Autodesk Fusion 360 part; units mm, degrees
(part 2 of 25)
sketch "Top SIlkscreen" plane through (0, 0, 0) normal (0, 0, 1) x (1, 0, 0)
  line L0 (55.2958, 9.3303) -> (56.4642, 9.7197)
  arc A0 (55.2878, 9.3544) -> (55.3038, 9.3062) centre (55.2958, 9.3303) ccw
  arc A1 (52.7304, 13.311) -> (52.7812, 13.311) centre (52.7558, 13.311) ccw
  line L1 (56.1721, 9.6224) -> (56.1721, 9.0382)
  arc A2 (56.4722, 9.6956) -> (56.4562, 9.7438) centre (56.4642, 9.7197) ccw
  arc A3 (53.6646, 12.8425) -> (53.6646, 12.7917) centre (53.6646, 12.8171) ccw
  arc A4 (53.9242, 13.2856) -> (53.9242, 13.3364) centre (53.9242, 13.311) ccw
  arc A5 (53.9242, 10.5777) -> (53.9242, 10.6285) centre (53.9242, 10.6031) ccw
  arc A6 (53.6392, 10.1487) -> (53.69, 10.1487) centre (53.6646, 10.1487) ccw
  arc A7 (52.6347, 11.7855) -> (52.6173, 11.7377) centre (52.626, 11.7616) ccw
  arc A8 (53.8988, 12.5575) -> (53.9496, 12.5575) centre (53.9242, 12.5575) ccw
  arc A9 (52.7304, 12.4601) -> (52.7812, 12.4601) centre (52.7558, 12.4601) ccw
  line L2 (53.4049, 10.6031) -> (53.9242, 10.6031)
  arc A10 (53.7619, 12.168) -> (53.9242, 12.5575) centre (53.3757, 12.5575) ccw
  arc A11 (53.8988, 13.6356) -> (53.9496, 13.6356) centre (53.9242, 13.6356) ccw
  arc A12 (52.7638, 14.8408) -> (52.7478, 14.7926) centre (52.7558, 14.8167) ccw
  line L3 (53.9242, 13.6356) -> (53.9242, 13.311)
  arc A13 (52.8532, 12.7522) -> (52.7558, 12.4601) centre (53.2426, 12.4601) ccw
  arc A14 (53.0154, 12.1751) -> (53.0154, 12.2259) centre (53.0154, 12.2005) ccw
  arc A15 (53.6646, 12.8171) -> (53.4374, 12.6873) centre (53.6646, 12.5534) ccw
  line L4 (52.7558, 14.8167) -> (53.9242, 15.2061)
  arc A16 (53.9162, 14.4031) -> (53.9322, 14.4513) centre (53.9242, 14.4272) ccw
  arc A17 (53.69, 10.7978) -> (53.6392, 10.7978) centre (53.6646, 10.7978) ccw
  arc A18 (54.0453, 11.2184) -> (54.0627, 11.2662) centre (54.054, 11.2423) ccw
  arc A19 (53.0804, 13.9347) -> (53.0804, 13.9855) centre (53.0804, 13.9601) ccw
  arc A20 (53.8988, 13.311) -> (53.9496, 13.311) centre (53.9242, 13.311) ccw
  line L5 (56.4642, 8.9408) -> (55.2958, 9.3303)
  arc A21 (52.7812, 13.6356) -> (52.7304, 13.6356) centre (52.7558, 13.6356) ccw
  line L6 (53.9242, 14.4272) -> (52.7558, 14.8167)
  line L7 (53.6321, 15.1088) -> (53.6321, 14.5246)
  arc A22 (52.8735, 12.737) -> (52.8328, 12.7674) centre (52.8531, 12.7522) ccw
  arc A23 (53.0804, 13.9855) -> (53.0804, 13.9347) centre (53.0804, 13.9601) ccw
  arc A24 (55.3038, 9.3544) -> (55.2878, 9.3062) centre (55.2958, 9.3303) ccw
  arc A25 (53.744, 12.186) -> (53.7798, 12.15) centre (53.7619, 12.168) ccw
  arc A26 (53.0154, 12.2005) -> (53.2426, 12.3303) centre (53.0154, 12.4642) ccw
  arc A27 (52.7628, 10.4328) -> (52.7488, 10.3839) centre (52.7558, 10.4084) ccw
  arc A28 (52.7558, 12.4601) -> (53.0154, 12.2005) centre (53.0154, 12.4601) ccw
  line L8 (53.9242, 13.311) -> (52.7558, 13.311)
  arc A29 (53.2203, 12.3424) -> (53.2649, 12.3181) centre (53.2426, 12.3302) ccw
  arc A30 (52.7812, 12.4601) -> (52.7304, 12.4601) centre (52.7558, 12.4601) ccw
  arc A31 (53.4049, 10.6285) -> (53.4049, 10.5777) centre (53.4049, 10.6031) ccw
  arc A32 (53.0154, 12.2259) -> (53.0154, 12.1751) centre (53.0154, 12.2005) ccw
  arc A33 (52.7304, 13.6356) -> (52.7812, 13.6356) centre (52.7558, 13.6356) ccw
  line L9 (53.0804, 13.9601) -> (53.5996, 13.9601)
  arc A34 (53.9496, 12.5575) -> (53.8988, 12.5575) centre (53.9242, 12.5575) ccw
  arc A35 (53.5996, 13.9855) -> (53.5996, 13.9347) centre (53.5996, 13.9601) ccw
  arc A36 (53.5996, 13.9347) -> (53.5996, 13.9855) centre (53.5996, 13.9601) ccw
  line L10 (53.4374, 12.6873) -> (53.2426, 12.3303)
  arc A37 (53.0804, 13.9601) -> (52.7558, 13.6356) centre (53.0804, 13.6355) ccw
  arc A38 (53.9242, 13.6356) -> (53.5996, 13.9601) centre (53.5996, 13.6355) ccw
  arc A39 (53.9242, 12.5575) -> (53.6646, 12.8171) centre (53.6646, 12.5575) ccw
  arc A40 (53.2645, 12.3174) -> (53.2208, 12.3432) centre (53.2427, 12.3303) ccw
  arc A41 (53.4155, 12.7002) -> (53.4593, 12.6744) centre (53.4374, 12.6873) ccw
  arc A42 (53.4597, 12.6751) -> (53.4151, 12.6995) centre (53.4374, 12.6873) ccw
  arc A43 (53.9322, 15.182) -> (53.9162, 15.2302) centre (53.9242, 15.2061) ccw
  arc A44 (56.4562, 8.9167) -> (56.4722, 8.9649) centre (56.4642, 8.9408) ccw
  arc A45 (53.6646, 12.7917) -> (53.6646, 12.8425) centre (53.6646, 12.8171) ccw
  arc A46 (52.7478, 14.8408) -> (52.7638, 14.7926) centre (52.7558, 14.8167) ccw
  line L11 (54.054, 11.2423) -> (52.626, 11.7616)
  arc A47 (53.6575, 15.1088) -> (53.6067, 15.1088) centre (53.6321, 15.1088) ccw
  line L12 (52.7558, 13.311) -> (52.7558, 13.6356)
  arc A48 (52.7558, 13.3364) -> (52.7558, 13.2856) centre (52.7558, 13.311) ccw
  arc A49 (53.6067, 14.5246) -> (53.6575, 14.5246) centre (53.6321, 14.5246) ccw
  arc A50 (53.9496, 13.6356) -> (53.8988, 13.6356) centre (53.9242, 13.6356) ccw
  arc A51 (55.3212, 12.4601) -> (55.2704, 12.4601) centre (55.2958, 12.4601) ccw
  arc A52 (56.4642, 10.5382) -> (56.2046, 10.7978) centre (56.2046, 10.5382) ccw
  arc A53 (56.2046, 10.7724) -> (56.2046, 10.8232) centre (56.2046, 10.7978) ccw
  arc A54 (41.0619, 54.9233) -> (41.2242, 55.1504) centre (40.9841, 55.1504) ccw
  arc A55 (56.2046, 12.8425) -> (56.2046, 12.7917) centre (56.2046, 12.8171) ccw
  arc A56 (41.0537, 54.9473) -> (41.0702, 54.8992) centre (41.062, 54.9233) ccw
  line L13 (56.4642, 10.1487) -> (56.4642, 10.5382)
  arc A57 (56.4388, 12.5575) -> (56.4896, 12.5575) centre (56.4642, 12.5575) ccw
  arc A58 (41.1988, 55.1504) -> (41.2496, 55.1504) centre (41.2242, 55.1504) ccw
  arc A59 (55.2958, 10.1741) -> (55.2958, 10.1233) centre (55.2958, 10.1487) ccw
  arc A60 (40.64, 54.8513) -> (40.64, 54.8005) centre (40.64, 54.8259) ccw
  arc A61 (56.0747, 10.7724) -> (56.0747, 10.8232) centre (56.0747, 10.7978) ccw
  arc A62 (41.2242, 55.1504) -> (41.0619, 55.3776) centre (40.984, 55.1504) ccw
  arc A63 (41.0508, 55.3548) -> (41.0731, 55.4005) centre (41.0619, 55.3777) ccw
  arc A64 (55.7897, 10.1487) -> (55.8405, 10.1487) centre (55.8151, 10.1487) ccw
  arc A65 (55.3212, 10.7978) -> (55.2704, 10.7978) centre (55.2958, 10.7978) ccw
  arc A66 (56.4388, 10.1487) -> (56.4896, 10.1487) centre (56.4642, 10.1487) ccw
  line L14 (55.2958, 10.1487) -> (55.2958, 10.7978)
  arc A67 (56.4642, 12.5575) -> (56.2046, 12.8171) centre (56.2046, 12.5575) ccw
  arc A68 (34.8822, 28.7456) -> (34.8662, 28.7938) centre (34.8742, 28.7697) ccw
  arc A69 (40.64, 55.5004) -> (40.64, 55.4496) centre (40.64, 55.475) ccw
  arc A70 (56.4896, 10.5382) -> (56.4388, 10.5382) centre (56.4642, 10.5382) ccw
  arc A71 (56.3019, 12.168) -> (56.4642, 12.5575) centre (55.9157, 12.5575) ccw
  arc A72 (55.1747, 11.7855) -> (55.1573, 11.7377) centre (55.166, 11.7616) ccw
  arc A73 (55.5554, 12.1751) -> (55.5554, 12.2259) centre (55.5554, 12.2005) ccw
  arc A74 (56.2046, 10.8232) -> (56.2046, 10.7724) centre (56.2046, 10.7978) ccw
  arc A75 (55.8405, 10.5382) -> (55.7897, 10.5382) centre (55.8151, 10.5382) ccw
  arc A76 (41.0702, 55.4017) -> (41.0537, 55.3536) centre (41.0619, 55.3777) ccw
  arc A77 (55.8151, 10.1233) -> (55.8151, 10.1741) centre (55.8151, 10.1487) ccw
  line L15 (56.594, 11.2423) -> (55.166, 11.7616)
  line L16 (55.8151, 10.5382) -> (55.8151, 10.1487)
  arc A78 (40.9487, 54.871) -> (40.9804, 54.9106) centre (40.9646, 54.8908) ccw
  line L17 (40.9646, 54.8908) -> (40.3154, 55.4101)
  arc A79 (41.0619, 55.3776) -> (40.64, 55.475) centre (40.6399, 54.5123) ccw
  arc A80 (40.3313, 55.4299) -> (40.2996, 55.3903) centre (40.3154, 55.4101) ccw
  line L18 (43.7642, 52.5018) -> (42.5958, 52.5018)
  line L19 (42.5958, 52.5018) -> (42.5958, 52.8264)
  arc A81 (56.0747, 10.8232) -> (56.0747, 10.7724) centre (56.0747, 10.7978) ccw
  arc A82 (55.2704, 10.1487) -> (55.3212, 10.1487) centre (55.2958, 10.1487) ccw
  line L20 (56.2046, 10.7978) -> (56.0747, 10.7978)
  arc A83 (56.1975, 9.6224) -> (56.1467, 9.6224) centre (56.1721, 9.6224) ccw
  arc A84 (56.0747, 10.7978) -> (55.8151, 10.5382) centre (56.0747, 10.5382) ccw
  line L21 (55.8151, 10.1487) -> (55.2958, 10.1487)
  arc A85 (55.2958, 12.4601) -> (55.5554, 12.2005) centre (55.5554, 12.4601) ccw
  arc A86 (55.3932, 12.7522) -> (55.2958, 12.4601) centre (55.7826, 12.4601) ccw
  arc A87 (56.284, 12.186) -> (56.3198, 12.15) centre (56.3019, 12.168) ccw
  line L22 (26.6051, 29.6644) -> (26.6051, 29.2749)
  arc A88 (56.4896, 12.5575) -> (56.4388, 12.5575) centre (56.4642, 12.5575) ccw
  arc A89 (40.64, 55.4496) -> (40.64, 55.5004) centre (40.64, 55.475) ccw
  arc A90 (40.2069, 55.4005) -> (40.2292, 55.3548) centre (40.218, 55.3777) ccw
  arc A91 (41.0731, 54.9004) -> (41.0508, 54.9461) centre (41.062, 54.9233) ccw
  arc A92 (56.4388, 10.5382) -> (56.4896, 10.5382) centre (56.4642, 10.5382) ccw
  line L23 (43.9972, 30.4165) -> (44.6322, 30.4165)
  arc A93 (40.0304, 55.1504) -> (40.0812, 55.1504) centre (40.0558, 55.1504) ccw
  arc A94 (41.2496, 55.1504) -> (41.1988, 55.1504) centre (41.2242, 55.1504) ccw
  line L24 (29.1451, 28.4452) -> (29.1451, 28.6399)
  arc A95 (56.5853, 11.2184) -> (56.6027, 11.2662) centre (56.594, 11.2423) ccw
  arc A96 (47.9679, 10.7724) -> (47.9679, 10.8232) centre (47.9679, 10.7978) ccw
  line L25 (26.6051, 29.2749) -> (26.0858, 29.2749)
  arc A97 (40.64, 55.475) -> (40.2181, 55.3776) centre (40.6401, 54.5123) ccw
  arc A98 (56.1467, 9.0382) -> (56.1975, 9.0382) centre (56.1721, 9.0382) ccw
  arc A99 (40.64, 54.8259) -> (41.0619, 54.9233) centre (40.6399, 55.7886) ccw
  arc A100 (55.7897, 10.5382) -> (55.8405, 10.5382) centre (55.8151, 10.5382) ccw
  arc A101 (45.8526, 54.3066) -> (45.8526, 54.3574) centre (45.8526, 54.332) ccw
  arc A102 (42.9204, 53.1509) -> (42.5958, 52.8264) centre (42.9204, 52.8263) ccw
  line L26 (43.7642, 52.8264) -> (43.7642, 52.5018)
  arc A103 (45.8526, 53.7083) -> (45.8526, 53.6575) centre (45.8526, 53.6829) ccw
  arc A104 (45.8526, 53.1763) -> (45.8526, 53.1255) centre (45.8526, 53.1509) ccw
  arc A105 (45.8526, 54.3574) -> (45.8526, 54.3066) centre (45.8526, 54.332) ccw
  arc A106 (45.2684, 53.7478) -> (45.2684, 54.2671) centre (45.2684, 54.0075) ccw
  arc A107 (43.7388, 52.8264) -> (43.7896, 52.8264) centre (43.7642, 52.8264) ccw
  arc A108 (45.3334, 53.1255) -> (45.3334, 53.1763) centre (45.3334, 53.1509) ccw
  arc A109 (44.9834, 52.5018) -> (45.0342, 52.5018) centre (45.0088, 52.5018) ccw
  arc A110 (45.2684, 54.2925) -> (45.2684, 54.2417) centre (45.2684, 54.2671) ccw
  arc A111 (45.2684, 53.7732) -> (45.2684, 53.7224) centre (45.2684, 53.7478) ccw
  arc A112 (42.9853, 53.6829) -> (43.2449, 53.9425) centre (42.9853, 53.9425) ccw
  arc A113 (42.9204, 53.6575) -> (42.9204, 53.7083) centre (42.9204, 53.6829) ccw
  arc A114 (42.9204, 54.3066) -> (42.9204, 54.3574) centre (42.9204, 54.332) ccw
  arc A115 (43.2449, 54.3066) -> (43.2449, 54.3574) centre (43.2449, 54.332) ccw
  arc A116 (43.2449, 54.3574) -> (43.2449, 54.3066) centre (43.2449, 54.332) ccw
  arc A117 (42.9204, 53.7083) -> (42.9204, 53.6575) centre (42.9204, 53.6829) ccw
  arc A118 (42.9853, 53.6575) -> (42.9853, 53.7083) centre (42.9853, 53.6829) ccw
  arc A119 (42.9204, 53.1763) -> (42.9204, 53.1255) centre (42.9204, 53.1509) ccw
  arc A120 (43.2703, 53.9425) -> (43.2195, 53.9425) centre (43.2449, 53.9425) ccw
  arc A121 (42.5704, 52.8264) -> (42.6212, 52.8264) centre (42.5958, 52.8264) ccw
  arc A122 (43.2703, 54.332) -> (43.2195, 54.332) centre (43.2449, 54.332) ccw
  line L27 (42.9853, 53.6829) -> (42.9204, 53.6829)
  line L28 (42.9204, 54.332) -> (43.2449, 54.332)
  arc A123 (43.7642, 53.8127) -> (43.2449, 54.332) centre (43.2449, 53.8127) ccw
  arc A124 (46.1772, 52.4764) -> (46.1772, 52.5272) centre (46.1772, 52.5018) ccw
  arc A125 (45.0342, 52.8264) -> (44.9834, 52.8264) centre (45.0088, 52.8264) ccw
  line L29 (42.9204, 53.1509) -> (43.4396, 53.1509)
  arc A126 (45.0088, 52.5272) -> (45.0088, 52.4764) centre (45.0088, 52.5018) ccw
  line L30 (45.0088, 52.5018) -> (45.0088, 52.8264)
  line L31 (45.3334, 53.1509) -> (45.8526, 53.1509)
  arc A127 (42.9204, 54.332) -> (42.9204, 53.6829) centre (42.9204, 54.0074) ccw
  arc A128 (43.7388, 52.5018) -> (43.7896, 52.5018) centre (43.7642, 52.5018) ccw
  arc A129 (45.3334, 53.1763) -> (45.3334, 53.1255) centre (45.3334, 53.1509) ccw
  arc A130 (46.1518, 52.8264) -> (46.2026, 52.8264) centre (46.1772, 52.8264) ccw
  arc A131 (43.7642, 52.8264) -> (43.4396, 53.1509) centre (43.4396, 52.8263) ccw
  line L32 (46.1772, 52.8264) -> (46.1772, 52.5018)
  arc A132 (45.3334, 53.1509) -> (45.0088, 52.8264) centre (45.3334, 52.8263) ccw
  arc A133 (45.8526, 53.6575) -> (45.8526, 53.7083) centre (45.8526, 53.6829) ccw
  arc A134 (43.7896, 52.8264) -> (43.7388, 52.8264) centre (43.7642, 52.8264) ccw
  arc A135 (46.1772, 52.8264) -> (45.8526, 53.1509) centre (45.8526, 52.8263) ccw
  arc A136 (42.9853, 53.7083) -> (42.9853, 53.6575) centre (42.9853, 53.6829) ccw
  arc A137 (45.2684, 54.2417) -> (45.2684, 54.2925) centre (45.2684, 54.2671) ccw
  arc A138 (45.2684, 53.7224) -> (45.2684, 53.7732) centre (45.2684, 53.7478) ccw
  arc A139 (42.5704, 52.5018) -> (42.6212, 52.5018) centre (42.5958, 52.5018) ccw
  arc A140 (43.4396, 53.1255) -> (43.4396, 53.1763) centre (43.4396, 53.1509) ccw
  arc A141 (43.2195, 53.9425) -> (43.2703, 53.9425) centre (43.2449, 53.9425) ccw
  line L33 (46.1772, 52.5018) -> (45.0088, 52.5018)
  arc A142 (45.8526, 53.1255) -> (45.8526, 53.1763) centre (45.8526, 53.1509) ccw
  arc A143 (42.5958, 52.5272) -> (42.5958, 52.4764) centre (42.5958, 52.5018) ccw
  arc A144 (42.9204, 53.1255) -> (42.9204, 53.1763) centre (42.9204, 53.1509) ccw
  arc A145 (42.9204, 54.3574) -> (42.9204, 54.3066) centre (42.9204, 54.332) ccw
  arc A146 (46.1518, 52.5018) -> (46.2026, 52.5018) centre (46.1772, 52.5018) ccw
  arc A147 (42.6212, 52.8264) -> (42.5704, 52.8264) centre (42.5958, 52.8264) ccw
  arc A148 (43.7388, 53.8127) -> (43.7896, 53.8127) centre (43.7642, 53.8127) ccw
  arc A149 (43.4396, 53.1763) -> (43.4396, 53.1255) centre (43.4396, 53.1509) ccw
  line L34 (43.2449, 54.332) -> (43.2449, 53.9425)
  arc A150 (44.9834, 52.8264) -> (45.0342, 52.8264) centre (45.0088, 52.8264) ccw
  arc A151 (43.7642, 52.4764) -> (43.7642, 52.5272) centre (43.7642, 52.5018) ccw
  arc A152 (45.8526, 53.6829) -> (45.8526, 54.332) centre (45.8526, 54.0074) ccw
  arc A153 (46.2026, 52.8264) -> (46.1518, 52.8264) centre (46.1772, 52.8264) ccw
  arc A154 (45.8526, 54.332) -> (45.8526, 53.6829) centre (45.8526, 54.0074) ccw
  arc A155 (45.2684, 54.2671) -> (45.2684, 53.7478) centre (45.2684, 54.0075) ccw
  arc A156 (51.0596, 54.3066) -> (51.0596, 54.3574) centre (51.0596, 54.332) ccw
  arc A157 (48.0004, 53.189) -> (48.0004, 53.2398) centre (48.0004, 53.2144) ccw
  line L35 (47.6758, 53.7464) -> (47.6758, 54.3955)
  arc A158 (50.5404, 53.1509) -> (50.2158, 52.8264) centre (50.5404, 52.8263) ccw
  arc A159 (47.6758, 52.5907) -> (47.6758, 52.5399) centre (47.6758, 52.5653) ccw
  arc A160 (50.2412, 54.2022) -> (50.1904, 54.2022) centre (50.2158, 54.2022) ccw
  arc A161 (51.0596, 53.6575) -> (51.0596, 53.7083) centre (51.0596, 53.6829) ccw
  arc A162 (47.6504, 53.7464) -> (47.7012, 53.7464) centre (47.6758, 53.7464) ccw
  line L36 (53.9242, 52.5018) -> (52.7558, 52.5018)
  arc A163 (47.7012, 52.8899) -> (47.6504, 52.8899) centre (47.6758, 52.8899) ccw
  arc A164 (47.6504, 52.5653) -> (47.7012, 52.5653) centre (47.6758, 52.5653) ccw
  arc A165 (48.5196, 53.189) -> (48.5196, 53.2398) centre (48.5196, 53.2144) ccw
  arc A166 (48.8188, 52.8899) -> (48.8696, 52.8899) centre (48.8442, 52.8899) ccw
  arc A167 (50.5404, 53.1763) -> (50.5404, 53.1255) centre (50.5404, 53.1509) ccw
  arc A168 (48.0004, 53.2144) -> (47.6758, 52.8899) centre (48.0004, 52.8898) ccw
  line L37 (51.3842, 52.8264) -> (51.3842, 52.5018)
  arc A169 (51.0596, 53.1763) -> (51.0596, 53.1255) centre (51.0596, 53.1509) ccw
  arc A170 (51.3588, 52.5018) -> (51.4096, 52.5018) centre (51.3842, 52.5018) ccw
  arc A171 (51.3842, 52.8264) -> (51.0596, 53.1509) centre (51.0596, 52.8263) ccw
  arc A172 (47.6826, 54.42) -> (47.669, 54.371) centre (47.6758, 54.3955) ccw
  arc A173 (50.1904, 52.8264) -> (50.2412, 52.8264) centre (50.2158, 52.8264) ccw
  line L38 (47.6758, 54.3955) -> (48.8442, 54.071)
  line L39 (50.5404, 53.1509) -> (51.0596, 53.1509)
  arc A174 (51.0596, 53.1255) -> (51.0596, 53.1763) centre (51.0596, 53.1509) ccw
  arc A175 (51.4096, 52.8264) -> (51.3588, 52.8264) centre (51.3842, 52.8264) ccw
  line L40 (48.8442, 52.8899) -> (48.8442, 52.5653)
  arc A176 (50.9947, 54.332) -> (50.7351, 54.0724) centre (50.9947, 54.0724) ccw
  arc A177 (50.7605, 54.0724) -> (50.7097, 54.0724) centre (50.7351, 54.0724) ccw
  arc A178 (47.7012, 54.3955) -> (47.6504, 54.3955) centre (47.6758, 54.3955) ccw
  arc A179 (50.9947, 54.3066) -> (50.9947, 54.3574) centre (50.9947, 54.332) ccw
  line L41 (50.9947, 54.332) -> (51.0596, 54.332)
  arc A180 (51.0596, 53.6829) -> (51.0596, 54.332) centre (51.0596, 54.0074) ccw
  arc A181 (47.6504, 52.8899) -> (47.7012, 52.8899) centre (47.6758, 52.8899) ccw
  line L42 (48.0004, 53.2144) -> (48.5196, 53.2144)
  arc A182 (48.5196, 53.2398) -> (48.5196, 53.189) centre (48.5196, 53.2144) ccw
  arc A183 (51.3842, 52.4764) -> (51.3842, 52.5272) centre (51.3842, 52.5018) ccw
  arc A184 (48.8374, 54.0465) -> (48.851, 54.0954) centre (48.8442, 54.0709) ccw
  arc A185 (51.3588, 52.8264) -> (51.4096, 52.8264) centre (51.3842, 52.8264) ccw
  arc A186 (48.8442, 52.8899) -> (48.5196, 53.2144) centre (48.5196, 52.8898) ccw
  arc A187 (51.0596, 54.3574) -> (51.0596, 54.3066) centre (51.0596, 54.332) ccw
  line L43 (50.2158, 52.5018) -> (50.2158, 52.8264)
  arc A188 (50.7351, 53.7083) -> (50.7351, 53.6575) centre (50.7351, 53.6829) ccw
  arc A189 (50.5404, 53.1255) -> (50.5404, 53.1763) centre (50.5404, 53.1509) ccw
  arc A190 (50.7351, 53.6575) -> (50.7351, 53.7083) centre (50.7351, 53.6829) ccw
  arc A191 (50.2158, 54.2022) -> (50.7351, 53.6829) centre (50.7351, 54.2022) ccw
  arc A192 (47.6758, 53.7718) -> (47.6758, 53.721) centre (47.6758, 53.7464) ccw
  arc A193 (50.2158, 52.5272) -> (50.2158, 52.4764) centre (50.2158, 52.5018) ccw
  arc A194 (50.1904, 52.5018) -> (50.2412, 52.5018) centre (50.2158, 52.5018) ccw
  arc A195 (50.7097, 54.0724) -> (50.7605, 54.0724) centre (50.7351, 54.0724) ccw
  arc A196 (50.9947, 54.3574) -> (50.9947, 54.3066) centre (50.9947, 54.332) ccw
  line L44 (47.6758, 52.5653) -> (47.6758, 52.8899)
  arc A197 (48.8696, 52.8899) -> (48.8188, 52.8899) centre (48.8442, 52.8899) ccw
  arc A198 (48.8442, 52.5399) -> (48.8442, 52.5907) centre (48.8442, 52.5653) ccw
  arc A199 (47.8056, 53.721) -> (47.8056, 53.7718) centre (47.8056, 53.7464) ccw
  line L45 (47.8056, 53.7464) -> (47.6758, 53.7464)
  arc A200 (48.0004, 53.2398) -> (48.0004, 53.189) centre (48.0004, 53.2144) ccw
  line L46 (51.3842, 52.5018) -> (50.2158, 52.5018)
  line L47 (48.8442, 52.5653) -> (47.6758, 52.5653)
  arc A201 (50.2412, 52.8264) -> (50.1904, 52.8264) centre (50.2158, 52.8264) ccw
  arc A202 (48.8188, 52.5653) -> (48.8696, 52.5653) centre (48.8442, 52.5653) ccw
  arc A203 (50.7097, 53.6829) -> (50.7605, 53.6829) centre (50.7351, 53.6829) ccw
  line L48 (50.7351, 53.6829) -> (50.7351, 54.0724)
  arc A204 (51.0596, 53.7083) -> (51.0596, 53.6575) centre (51.0596, 53.6829) ccw
  line L49 (51.0596, 53.6829) -> (50.7351, 53.6829)
  line L50 (56.4642, 52.5018) -> (55.2958, 52.5018)
  arc A205 (40.2263, 55.3536) -> (40.2098, 55.4017) centre (40.2181, 55.3776) ccw
  arc A206 (53.5996, 53.1255) -> (53.5996, 53.1763) centre (53.5996, 53.1509) ccw
  arc A207 (53.9496, 52.8264) -> (53.8988, 52.8264) centre (53.9242, 52.8264) ccw
  arc A208 (54.6885, 2.4638) -> (54.6885, 2.5146) centre (54.6885, 2.4892) ccw
  arc A209 (55.2704, 52.5018) -> (55.3212, 52.5018) centre (55.2958, 52.5018) ccw
  arc A210 (55.6204, 53.1255) -> (55.6204, 53.1763) centre (55.6204, 53.1509) ccw
  arc A211 (53.0804, 53.1509) -> (52.7558, 52.8264) centre (53.0804, 52.8263) ccw
  arc A212 (56.4388, 52.8264) -> (56.4896, 52.8264) centre (56.4642, 52.8264) ccw
  line L51 (52.7558, 52.5018) -> (52.7558, 52.8264)
  arc A213 (53.9242, 52.4764) -> (53.9242, 52.5272) centre (53.9242, 52.5018) ccw
  line L52 (26.0858, 30.353) -> (27.2542, 30.7425)
  arc A214 (54.4542, 1.5804) -> (54.4034, 1.5804) centre (54.4288, 1.5804) ccw
  line L53 (53.6646, 54.332) -> (53.5347, 54.332)
  arc A215 (26.8647, 29.8986) -> (26.8647, 29.9494) centre (26.8647, 29.924) ccw
  arc A216 (53.6646, 54.3066) -> (53.6646, 54.3574) centre (53.6646, 54.332) ccw
  arc A217 (53.5347, 54.3574) -> (53.5347, 54.3066) centre (53.5347, 54.332) ccw
  arc A218 (53.5347, 54.332) -> (53.2751, 54.0724) centre (53.5347, 54.0724) ccw
  arc A219 (53.5347, 54.3066) -> (53.5347, 54.3574) centre (53.5347, 54.332) ccw
  arc A220 (53.5996, 53.1763) -> (53.5996, 53.1255) centre (53.5996, 53.1509) ccw
  arc A221 (53.8988, 54.0724) -> (53.9496, 54.0724) centre (53.9242, 54.0724) ccw
  arc A222 (52.7304, 52.8264) -> (52.7812, 52.8264) centre (52.7558, 52.8264) ccw
  arc A223 (53.9242, 54.0724) -> (53.6646, 54.332) centre (53.6646, 54.0724) ccw
  arc A224 (53.8988, 53.6829) -> (53.9496, 53.6829) centre (53.9242, 53.6829) ccw
  arc A225 (52.7558, 53.7083) -> (52.7558, 53.6575) centre (52.7558, 53.6829) ccw
  arc A226 (34.8662, 27.9667) -> (34.8822, 28.0149) centre (34.8742, 27.9908) ccw
  arc A227 (53.2497, 53.6829) -> (53.3005, 53.6829) centre (53.2751, 53.6829) ccw
  arc A228 (53.3005, 54.0724) -> (53.2497, 54.0724) centre (53.2751, 54.0724) ccw
  arc A229 (53.0804, 53.1255) -> (53.0804, 53.1763) centre (53.0804, 53.1509) ccw
  arc A230 (53.2751, 53.6575) -> (53.2751, 53.7083) centre (53.2751, 53.6829) ccw
  arc A231 (52.7812, 54.332) -> (52.7304, 54.332) centre (52.7558, 54.332) ccw
  arc A232 (56.4642, 52.4764) -> (56.4642, 52.5272) centre (56.4642, 52.5018) ccw
  arc A233 (51.1246, 29.8986) -> (51.1246, 29.9494) centre (51.1246, 29.924) ccw
  line L54 (29.7942, 28.6399) -> (29.7942, 28.2504)
  arc A234 (52.7812, 52.8264) -> (52.7304, 52.8264) centre (52.7558, 52.8264) ccw
  arc A235 (53.8988, 52.5018) -> (53.9496, 52.5018) centre (53.9242, 52.5018) ccw
  line L55 (53.9242, 52.8264) -> (53.9242, 52.5018)
  arc A236 (53.2497, 54.0724) -> (53.3005, 54.0724) centre (53.2751, 54.0724) ccw
  arc A237 (54.9481, 2.4638) -> (54.9481, 2.5146) centre (54.9481, 2.4892) ccw
  arc A238 (55.3212, 52.8264) -> (55.2704, 52.8264) centre (55.2958, 52.8264) ccw
  arc A239 (53.0804, 53.1763) -> (53.0804, 53.1255) centre (53.0804, 53.1509) ccw
  arc A240 (55.2958, 52.5272) -> (55.2958, 52.4764) centre (55.2958, 52.5018) ccw
  arc A241 (53.6646, 54.3574) -> (53.6646, 54.3066) centre (53.6646, 54.332) ccw
  arc A242 (55.6204, 53.1509) -> (55.2958, 52.8264) centre (55.6204, 52.8263) ccw
  arc A243 (55.2704, 52.8264) -> (55.3212, 52.8264) centre (55.2958, 52.8264) ccw
  arc A244 (52.7304, 52.5018) -> (52.7812, 52.5018) centre (52.7558, 52.5018) ccw
  arc A245 (53.8988, 52.8264) -> (53.9496, 52.8264) centre (53.9242, 52.8264) ccw
  arc A246 (53.9496, 54.0724) -> (53.8988, 54.0724) centre (53.9242, 54.0724) ccw
  line L56 (52.7558, 53.6829) -> (52.7558, 54.332)
  arc A247 (52.7304, 53.6829) -> (52.7812, 53.6829) centre (52.7558, 53.6829) ccw
  arc A248 (52.7558, 52.5272) -> (52.7558, 52.4764) centre (52.7558, 52.5018) ccw
  arc A249 (28.8854, 28.0162) -> (28.8854, 27.9654) centre (28.8854, 27.9908) ccw
  arc A250 (26.0778, 30.3771) -> (26.0938, 30.3289) centre (26.0858, 30.353) ccw
  line L57 (53.0804, 53.1509) -> (53.5996, 53.1509)
  arc A251 (26.0604, 29.2749) -> (26.1112, 29.2749) centre (26.0858, 29.2749) ccw
  arc A252 (33.7138, 28.4044) -> (33.6978, 28.3562) centre (33.7058, 28.3803) ccw
  arc A253 (53.9242, 52.8264) -> (53.5996, 53.1509) centre (53.5996, 52.8263) ccw
  line L58 (53.9242, 53.6829) -> (53.9242, 54.0724)
  line L59 (53.2751, 54.0724) -> (53.2751, 53.6829)
  arc A254 (29.8196, 28.6399) -> (29.7688, 28.6399) centre (29.7942, 28.6399) ccw
  line L60 (53.2751, 53.6829) -> (52.7558, 53.6829)
  line L61 (55.6204, 53.1509) -> (56.1396, 53.1509)
  line L62 (55.2958, 52.5018) -> (55.2958, 52.8264)
  arc A255 (56.1396, 53.1255) -> (56.1396, 53.1763) centre (56.1396, 53.1509) ccw
  arc A256 (61.5442, 52.8264) -> (61.2196, 53.1509) centre (61.2196, 52.8263) ccw
  arc A257 (56.23, 54.332) -> (56.1792, 54.332) centre (56.2046, 54.332) ccw
  arc A258 (58.1604, 53.1763) -> (58.1604, 53.1255) centre (58.1604, 53.1509) ccw
  line L63 (59.0042, 53.6829) -> (59.0042, 54.0075)
  arc A259 (59.0042, 54.0075) -> (58.3551, 54.0075) centre (58.6797, 54.0075) ccw
  arc A260 (55.3028, 53.967) -> (55.2888, 53.9181) centre (55.2958, 53.9426) ccw
  arc A261 (58.1604, 53.1509) -> (57.8358, 52.8264) centre (58.1604, 52.8263) ccw
  line L64 (56.2046, 53.6829) -> (56.2046, 54.332)
  arc A262 (58.3297, 54.0075) -> (58.3805, 54.0075) centre (58.3551, 54.0075) ccw
  arc A263 (57.8612, 52.8264) -> (57.8104, 52.8264) centre (57.8358, 52.8264) ccw
  arc A264 (57.8104, 53.6829) -> (57.8612, 53.6829) centre (57.8358, 53.6829) ccw
  arc A265 (56.1792, 53.6829) -> (56.23, 53.6829) centre (56.2046, 53.6829) ccw
  arc A266 (58.1604, 53.1255) -> (58.1604, 53.1763) centre (58.1604, 53.1509) ccw
  arc A267 (58.3551, 54.0724) -> (57.8358, 54.0724) centre (58.0954, 54.0724) ccw
  arc A268 (56.4896, 52.8264) -> (56.4388, 52.8264) centre (56.4642, 52.8264) ccw
  arc A269 (58.3297, 54.0724) -> (58.3805, 54.0724) centre (58.3551, 54.0724) ccw
  arc A270 (59.0296, 52.8264) -> (58.9788, 52.8264) centre (59.0042, 52.8264) ccw
  arc A271 (60.3758, 52.5272) -> (60.3758, 52.4764) centre (60.3758, 52.5018) ccw
  arc A272 (61.5442, 52.4764) -> (61.5442, 52.5272) centre (61.5442, 52.5018) ccw
  line L65 (61.5442, 52.5018) -> (60.3758, 52.5018)
  arc A273 (58.3297, 53.8127) -> (58.3805, 53.8127) centre (58.3551, 53.8127) ccw
  arc A274 (60.4012, 52.8264) -> (60.3504, 52.8264) centre (60.3758, 52.8264) ccw
  line L66 (59.0042, 52.5018) -> (57.8358, 52.5018)
  line L67 (55.9449, 54.1373) -> (56.4642, 54.1373)
  line L68 (59.0042, 52.8264) -> (59.0042, 52.5018)
  arc A275 (58.9788, 53.6829) -> (59.0296, 53.6829) centre (59.0042, 53.6829) ccw
  arc A276 (60.7004, 53.1509) -> (60.3758, 52.8264) centre (60.7004, 52.8263) ccw
  arc A277 (57.8104, 52.5018) -> (57.8612, 52.5018) centre (57.8358, 52.5018) ccw
  line L69 (60.7004, 53.1509) -> (61.2196, 53.1509)
  arc A278 (59.0042, 52.8264) -> (58.6796, 53.1509) centre (58.6796, 52.8263) ccw
  arc A279 (58.9788, 52.8264) -> (59.0296, 52.8264) centre (59.0042, 52.8264) ccw
  arc A280 (60.3504, 52.8264) -> (60.4012, 52.8264) centre (60.3758, 52.8264) ccw
  arc A281 (57.8612, 54.0724) -> (57.8104, 54.0724) centre (57.8358, 54.0724) ccw
  arc A282 (60.7004, 53.1763) -> (60.7004, 53.1255) centre (60.7004, 53.1509) ccw
  arc A283 (55.9449, 54.1627) -> (55.9449, 54.1119) centre (55.9449, 54.1373) ccw
  line L70 (57.8358, 52.5018) -> (57.8358, 52.8264)
  arc A284 (57.8104, 52.8264) -> (57.8612, 52.8264) centre (57.8358, 52.8264) ccw
  arc A285 (60.7004, 53.1255) -> (60.7004, 53.1763) centre (60.7004, 53.1509) ccw
  line L71 (58.3551, 54.0724) -> (58.3551, 53.8127)
  arc A286 (55.6204, 53.1763) -> (55.6204, 53.1255) centre (55.6204, 53.1509) ccw
  arc A287 (57.8358, 52.5272) -> (57.8358, 52.4764) centre (57.8358, 52.5018) ccw
  arc A288 (59.0042, 52.4764) -> (59.0042, 52.5272) centre (59.0042, 52.5018) ccw
  arc A289 (56.4642, 52.8264) -> (56.1396, 53.1509) centre (56.1396, 52.8263) ccw
  arc A290 (58.9788, 54.0075) -> (59.0296, 54.0075) centre (59.0042, 54.0075) ccw
  arc A291 (56.4388, 52.5018) -> (56.4896, 52.5018) centre (56.4642, 52.5018) ccw
  line L72 (56.4642, 52.8264) -> (56.4642, 52.5018)
  arc A292 (56.1976, 53.6585) -> (56.2115, 53.7073) centre (56.2045, 53.6829) ccw
  arc A293 (56.4642, 54.1119) -> (56.4642, 54.1627) centre (56.4642, 54.1373) ccw
  arc A294 (58.6796, 53.1255) -> (58.6796, 53.1763) centre (58.6796, 53.1509) ccw
  arc A295 (58.6796, 53.1763) -> (58.6796, 53.1255) centre (58.6796, 53.1509) ccw
  arc A296 (59.0296, 54.0075) -> (58.9788, 54.0075) centre (59.0042, 54.0075) ccw
  line L73 (58.1604, 53.1509) -> (58.6796, 53.1509)
  arc A297 (58.9788, 52.5018) -> (59.0296, 52.5018) centre (59.0042, 52.5018) ccw
  line L74 (55.2958, 53.9425) -> (56.2046, 53.6829)
  arc A298 (58.3805, 54.0724) -> (58.3297, 54.0724) centre (58.3551, 54.0724) ccw
  line L75 (57.8358, 53.6829) -> (57.8358, 54.0724)
  arc A299 (56.1396, 53.1763) -> (56.1396, 53.1255) centre (56.1396, 53.1509) ccw
  line L76 (60.3758, 52.5018) -> (60.3758, 52.8264)
  arc A300 (57.8104, 54.0724) -> (57.8612, 54.0724) centre (57.8358, 54.0724) ccw
  arc A301 (60.3504, 52.5018) -> (60.4012, 52.5018) centre (60.3758, 52.5018) ccw
  arc A302 (61.2196, 53.1255) -> (61.2196, 53.1763) centre (61.2196, 53.1509) ccw
  arc A303 (31.1578, 28.4044) -> (31.1738, 28.3562) centre (31.1658, 28.3803) ccw
  arc A304 (32.3422, 28.7456) -> (32.3262, 28.7938) centre (32.3342, 28.7697) ccw
  arc A305 (32.3262, 27.9667) -> (32.3422, 28.0149) centre (32.3342, 27.9908) ccw
  arc A306 (31.1738, 28.4044) -> (31.1578, 28.3562) centre (31.1658, 28.3803) ccw
  line L77 (31.4254, 29.1987) -> (31.1658, 29.5233)
  line L78 (61.5442, 53.6829) -> (61.5442, 54.332)
  line L79 (58.1604, 9.5899) -> (58.6796, 9.5899)
  arc A307 (60.6679, 54.3066) -> (60.6679, 54.3574) centre (60.6679, 54.332) ccw
  arc A308 (61.2196, 53.1763) -> (61.2196, 53.1255) centre (61.2196, 53.1509) ccw
  arc A309 (60.6276, 53.6587) -> (60.6433, 53.7071) centre (60.6355, 53.6829) ccw
  arc A310 (60.8951, 54.2346) -> (60.6679, 54.332) centre (60.6679, 54.0183) ccw
  line L80 (57.8358, 8.9408) -> (57.8358, 9.2654)
  arc A311 (61.5188, 52.5018) -> (61.5696, 52.5018) centre (61.5442, 52.5018) ccw
  arc A312 (60.6679, 54.332) -> (60.3758, 54.0399) centre (60.6679, 54.0399) ccw
  arc A313 (61.5696, 54.332) -> (61.5188, 54.332) centre (61.5442, 54.332) ccw
  line L81 (57.8358, 10.4465) -> (59.0042, 10.4465)
  line L82 (28.6258, 28.2504) -> (28.6258, 28.6399)
  arc A314 (57.8358, 8.9662) -> (57.8358, 8.9154) centre (57.8358, 8.9408) ccw
  line L83 (59.0042, 8.9408) -> (57.8358, 8.9408)
  arc A315 (57.8556, 10.4623) -> (57.816, 10.4306) centre (57.8358, 10.4465) ccw
  line L84 (59.0042, 10.1219) -> (59.0042, 10.771)
  arc A316 (32.3342, 29.4979) -> (32.3342, 29.5487) centre (32.3342, 29.5233) ccw
  arc A317 (60.4012, 54.0399) -> (60.3504, 54.0399) centre (60.3758, 54.0399) ccw
  arc A318 (60.6679, 54.3574) -> (60.6679, 54.3066) centre (60.6679, 54.332) ccw
  arc A319 (58.9788, 8.9408) -> (59.0296, 8.9408) centre (59.0042, 8.9408) ccw
  arc A320 (58.9788, 9.2654) -> (59.0296, 9.2654) centre (59.0042, 9.2654) ccw
  line L85 (61.5442, 52.8264) -> (61.5442, 52.5018)
  arc A321 (61.5696, 52.8264) -> (61.5188, 52.8264) centre (61.5442, 52.8264) ccw
  arc A322 (32.0167, 28.0882) -> (32.0675, 28.0882) centre (32.0421, 28.0882) ccw
  line L86 (32.3342, 29.1987) -> (32.3342, 29.8478)
  arc A323 (59.0042, 8.9154) -> (59.0042, 8.9662) centre (59.0042, 8.9408) ccw
  arc A324 (57.8358, 10.4718) -> (57.8358, 10.4211) centre (57.8358, 10.4465) ccw
  arc A325 (31.1658, 29.5487) -> (31.1658, 29.4979) centre (31.1658, 29.5233) ccw
  arc A326 (61.5188, 53.6829) -> (61.5696, 53.6829) centre (61.5442, 53.6829) ccw
  arc A327 (57.8612, 9.2654) -> (57.8104, 9.2654) centre (57.8358, 9.2654) ccw
  arc A328 (60.3758, 54.0399) -> (60.6354, 53.6829) centre (60.751, 54.0399) ccw
  arc A329 (61.5277, 53.6635) -> (61.5607, 53.7023) centre (61.5442, 53.6829) ccw
  line L87 (58.0954, 10.1219) -> (57.8358, 10.4465)
  arc A330 (59.0296, 9.2654) -> (58.9788, 9.2654) centre (59.0042, 9.2654) ccw
  arc A331 (58.1604, 9.5899) -> (57.8358, 9.2654) centre (58.1604, 9.2653) ccw
  arc A332 (60.3504, 54.0399) -> (60.4012, 54.0399) centre (60.3758, 54.0399) ccw
  arc A333 (58.6796, 9.5645) -> (58.6796, 9.6153) centre (58.6796, 9.5899) ccw
  arc A334 (59.0042, 10.4211) -> (59.0042, 10.4718) centre (59.0042, 10.4465) ccw
  arc A335 (61.5188, 52.8264) -> (61.5696, 52.8264) centre (61.5442, 52.8264) ccw
  arc A336 (60.9115, 54.254) -> (60.8786, 54.2153) centre (60.895, 54.2347) ccw
  line L88 (59.0042, 9.2654) -> (59.0042, 8.9408)
  arc A337 (31.4056, 29.1828) -> (31.4453, 29.2146) centre (31.4255, 29.1987) ccw
  arc A338 (31.1856, 29.5391) -> (31.146, 29.5074) centre (31.1658, 29.5233) ccw
  line L89 (34.8742, 27.9908) -> (33.7058, 28.3803)
  line L90 (31.1658, 29.5233) -> (32.3342, 29.5233)
  arc A339 (60.8767, 54.2171) -> (60.9135, 54.2522) centre (60.8951, 54.2346) ccw
  arc A340 (57.8104, 8.9408) -> (57.8612, 8.9408) centre (57.8358, 8.9408) ccw
  arc A341 (32.3088, 29.1987) -> (32.3596, 29.1987) centre (32.3342, 29.1987) ccw
  arc A342 (57.8104, 9.2654) -> (57.8612, 9.2654) centre (57.8358, 9.2654) ccw
  line L91 (34.5821, 28.6724) -> (34.5821, 28.0882)
  arc A343 (59.0042, 9.2654) -> (58.6796, 9.5899) centre (58.6796, 9.2653) ccw
  arc A344 (58.1604, 9.5645) -> (58.1604, 9.6153) centre (58.1604, 9.5899) ccw
  arc A345 (58.0756, 10.106) -> (58.1153, 10.1378) centre (58.0954, 10.1219) ccw
  line L92 (60.8951, 54.2346) -> (61.5442, 53.6829)
  arc A346 (32.3596, 29.8478) -> (32.3088, 29.8478) centre (32.3342, 29.8478) ccw
  arc A347 (58.6796, 9.6153) -> (58.6796, 9.5645) centre (58.6796, 9.5899) ccw
  line L93 (33.7058, 28.3803) -> (34.8742, 28.7697)
  arc A348 (58.1604, 9.6153) -> (58.1604, 9.5645) centre (58.1604, 9.5899) ccw
  arc A349 (32.0675, 28.6724) -> (32.0167, 28.6724) centre (32.0421, 28.6724) ccw
  arc A350 (28.6258, 29.2354) -> (28.6258, 29.1846) centre (28.6258, 29.21) ccw
  line L94 (70.485, 34.29) -> (52.07, 34.29)
  arc A351 (51.9938, 34.29) -> (52.1462, 34.29) centre (52.07, 34.29) ccw
  arc A352 (29.1705, 28.6399) -> (29.1197, 28.6399) centre (29.1451, 28.6399) ccw
  arc A353 (29.8065, 29.8369) -> (29.7819, 29.8813) centre (29.7942, 29.8591) ccw
  arc A354 (26.9946, 29.8986) -> (26.9946, 29.9494) centre (26.9946, 29.924) ccw
  arc A355 (29.7942, 52.6429) -> (29.7434, 52.6429) centre (29.7688, 52.6429) ccw
  arc A356 (29.7942, 30.4038) -> (29.7942, 30.4546) centre (29.7942, 30.4292) ccw
  arc A357 (29.7688, 52.2534) -> (30.0284, 51.9938) centre (30.0284, 52.2534) ccw
  arc A358 (28.9504, 31.0783) -> (28.6258, 30.7537) centre (28.9504, 30.7537) ccw
  line L95 (26.0858, 29.2749) -> (26.0858, 29.924)
  arc A359 (52.07, 40.7162) -> (52.07, 40.5638) centre (52.07, 40.64) ccw
  arc A360 (70.4088, 34.29) -> (70.5612, 34.29) centre (70.485, 34.29) ccw
  arc A361 (52.1462, 40.64) -> (51.9938, 40.64) centre (52.07, 40.64) ccw
  arc A362 (29.7942, 30.7537) -> (29.4696, 31.0783) centre (29.4696, 30.7537) ccw
  arc A363 (28.6004, 30.7537) -> (28.6512, 30.7537) centre (28.6258, 30.7537) ccw
  arc A364 (28.9504, 31.0529) -> (28.9504, 31.1037) centre (28.9504, 31.0783) ccw
  line L96 (31.1658, 28.3803) -> (32.3342, 28.7697)
  arc A365 (28.6512, 28.2504) -> (28.6004, 28.2504) centre (28.6258, 28.2504) ccw
  arc A366 (70.485, 40.5638) -> (70.485, 40.7162) centre (70.485, 40.64) ccw
  line L97 (29.7688, 52.2534) -> (29.7688, 52.6429)
  arc A367 (29.7942, 52.2534) -> (29.7434, 52.2534) centre (29.7688, 52.2534) ccw
  arc A368 (28.6135, 29.2322) -> (28.6381, 29.1878) centre (28.6258, 29.21) ccw
  arc A369 (28.6258, 30.4546) -> (28.6258, 30.4038) centre (28.6258, 30.4292) ccw
  line L98 (28.6258, 30.4292) -> (28.6258, 30.7537)
  arc A370 (28.9504, 31.1037) -> (28.9504, 31.0529) centre (28.9504, 31.0783) ccw
  arc A371 (70.485, 34.2138) -> (70.485, 34.3662) centre (70.485, 34.29) ccw
  line L99 (29.7688, 53.213) -> (30.9372, 53.8621)
  arc A372 (50.9947, 29.9494) -> (50.9947, 29.8986) centre (50.9947, 29.924) ccw
  arc A373 (28.6512, 30.7537) -> (28.6004, 30.7537) centre (28.6258, 30.7537) ccw
  arc A374 (29.4696, 31.1037) -> (29.4696, 31.0529) centre (29.4696, 31.0783) ccw
  arc A375 (29.7688, 53.2384) -> (29.7688, 53.1876) centre (29.7688, 53.213) ccw
  arc A376 (52.07, 34.3662) -> (52.07, 34.2138) centre (52.07, 34.29) ccw
  arc A377 (29.7688, 30.4292) -> (29.8196, 30.4292) centre (29.7942, 30.4292) ccw
  arc A378 (29.8196, 30.7537) -> (29.7688, 30.7537) centre (29.7942, 30.7537) ccw
  line L100 (52.07, 40.64) -> (70.485, 40.64)
  line L101 (33.6042, 52.5018) -> (32.4358, 52.5018)
  arc A379 (28.8854, 27.9654) -> (28.8854, 28.0162) centre (28.8854, 27.9908) ccw
  arc A380 (28.6004, 30.4292) -> (28.6512, 30.4292) centre (28.6258, 30.4292) ccw
  line L102 (29.7942, 30.4292) -> (28.6258, 30.4292)
  arc A381 (29.7688, 30.7537) -> (29.8196, 30.7537) centre (29.7942, 30.7537) ccw
  line L103 (32.3342, 27.9908) -> (31.1658, 28.3803)
  arc A382 (29.5346, 27.9654) -> (29.5346, 28.0162) centre (29.5346, 27.9908) ccw
  line L104 (52.07, 34.29) -> (52.07, 40.64)
  line L105 (32.0421, 28.6724) -> (32.0421, 28.0882)
  arc A383 (30.0284, 51.9684) -> (30.0284, 52.0192) centre (30.0284, 51.9938) ccw
  arc A384 (28.6258, 29.8845) -> (28.6258, 29.8337) centre (28.6258, 29.8591) ccw
  arc A385 (29.7434, 52.2534) -> (29.7942, 52.2534) centre (29.7688, 52.2534) ccw
  arc A386 (29.7942, 29.8337) -> (29.7942, 29.8845) centre (29.7942, 29.8591) ccw
  arc A387 (54.6885, 2.5146) -> (54.6885, 2.4638) centre (54.6885, 2.4892) ccw
  arc A388 (54.9481, 1.2954) -> (54.9481, 1.3462) centre (54.9481, 1.3208) ccw
  arc A389 (51.1246, 29.9494) -> (51.1246, 29.8986) centre (51.1246, 29.924) ccw
  line L106 (70.485, 40.64) -> (70.485, 34.29)
  arc A390 (29.7942, 29.1846) -> (29.7942, 29.2354) centre (29.7942, 29.21) ccw
  arc A391 (28.6258, 28.2504) -> (28.8854, 27.9908) centre (28.8854, 28.2504) ccw
  arc A392 (70.5612, 40.64) -> (70.4088, 40.64) centre (70.485, 40.64) ccw
  arc A393 (28.6004, 28.2504) -> (28.6512, 28.2504) centre (28.6258, 28.2504) ccw
  line L107 (29.7942, 30.7537) -> (29.7942, 30.4292)
  arc A394 (28.6512, 28.6399) -> (28.6004, 28.6399) centre (28.6258, 28.6399) ccw
  line L108 (29.7942, 29.8591) -> (28.6258, 29.8591)
  arc A395 (54.4542, 2.2296) -> (54.4034, 2.2296) centre (54.4288, 2.2296) ccw
  arc A396 (54.4288, 1.5804) -> (54.6885, 1.3208) centre (54.6885, 1.5805) ccw
  line L109 (29.7942, 29.21) -> (28.6258, 29.21)
  arc A397 (29.4696, 31.0529) -> (29.4696, 31.1037) centre (29.4696, 31.0783) ccw
  arc A398 (40.9646, 8.9662) -> (40.9646, 8.9154) centre (40.9646, 8.9408) ccw
  arc A399 (26.0096, 53.9355) -> (25.9588, 53.9355) centre (25.9842, 53.9355) ccw
  line L110 (25.9842, 52.8913) -> (24.8158, 53.2807)
  arc A400 (25.9842, 53.7803) -> (25.9842, 53.8311) centre (25.9842, 53.8057) ccw
  arc A401 (24.8412, 53.9355) -> (24.7904, 53.9355) centre (24.8158, 53.9355) ccw
  arc A402 (30.9372, 54.7567) -> (30.6126, 55.0813) centre (30.6126, 54.7567) ccw
  arc A403 (30.9372, 53.8367) -> (30.9372, 53.8875) centre (30.9372, 53.8621) ccw
  line L111 (28.6258, 29.21) -> (29.7942, 29.8591)
  arc A404 (25.9842, 54.4082) -> (25.9842, 54.459) centre (25.9842, 54.4336) ccw
  arc A405 (30.9372, 53.1876) -> (30.9372, 53.2384) centre (30.9372, 53.213) ccw
  arc A406 (30.0934, 55.1067) -> (30.0934, 55.0559) centre (30.0934, 55.0813) ccw
  line L112 (24.8158, 54.4336) -> (25.9842, 55.0827)
  arc A407 (30.9118, 54.4322) -> (30.9626, 54.4322) centre (30.9372, 54.4322) ccw
  line L113 (40.0558, 11.3792) -> (40.0558, 11.7037)
  arc A408 (26.5797, 29.2749) -> (26.6305, 29.2749) centre (26.6051, 29.2749) ccw
  line L114 (41.2242, 10.16) -> (40.0558, 10.16)
  line L115 (40.9646, 8.9408) -> (40.3154, 8.9408)
  arc A409 (40.3154, 8.9662) -> (40.3154, 8.9154) centre (40.3154, 8.9408) ccw
  line L116 (24.8158, 53.8057) -> (25.9842, 53.8057)
  line L117 (40.5751, 9.3952) -> (40.5751, 9.5899)
  line L118 (41.2242, 9.5899) -> (41.2242, 9.2004)
  arc A410 (40.0812, 9.5899) -> (40.0304, 9.5899) centre (40.0558, 9.5899) ccw
  arc A411 (40.9646, 8.9154) -> (40.9646, 8.9662) centre (40.9646, 8.9408) ccw
  arc A412 (40.3154, 8.9154) -> (40.3154, 8.9662) centre (40.3154, 8.9408) ccw
  line L119 (30.9372, 53.213) -> (29.7688, 53.213)
  line L120 (30.9372, 54.4322) -> (29.7688, 54.4322)
  arc A413 (30.9372, 54.4068) -> (30.9372, 54.4576) centre (30.9372, 54.4322) ccw
  arc A414 (29.7942, 54.7567) -> (29.7434, 54.7567) centre (29.7688, 54.7567) ccw
  line L121 (25.9842, 53.6758) -> (25.9842, 53.9355)
  line L122 (30.9372, 54.7567) -> (30.9372, 54.4322)
  arc A415 (25.9762, 52.8672) -> (25.9922, 52.9154) centre (25.9842, 52.8913) ccw
  arc A416 (24.8238, 53.3048) -> (24.8078, 53.2566) centre (24.8158, 53.2807) ccw
  arc A417 (30.9626, 54.7567) -> (30.9118, 54.7567) centre (30.9372, 54.7567) ccw
  arc A418 (40.5751, 9.6153) -> (40.5751, 9.5645) centre (40.5751, 9.5899) ccw
  arc A419 (24.7904, 53.6758) -> (24.8412, 53.6758) centre (24.8158, 53.6758) ccw
  line L123 (40.0558, 10.16) -> (41.2242, 10.8091)
  line L124 (30.9372, 53.8621) -> (29.7688, 53.8621)
  arc A420 (29.7434, 54.7567) -> (29.7942, 54.7567) centre (29.7688, 54.7567) ccw
  arc A421 (30.6126, 55.0559) -> (30.6126, 55.1067) centre (30.6126, 55.0813) ccw
  arc A422 (29.7688, 53.8875) -> (29.7688, 53.8367) centre (29.7688, 53.8621) ccw
  arc A423 (30.6126, 55.1067) -> (30.6126, 55.0559) centre (30.6126, 55.0813) ccw
  arc A424 (24.8158, 54.459) -> (24.8158, 54.4082) centre (24.8158, 54.4336) ccw
  arc A425 (30.9118, 54.7567) -> (30.9626, 54.7567) centre (30.9372, 54.7567) ccw
  arc A426 (30.0934, 55.0813) -> (29.7688, 54.7567) centre (30.0934, 54.7567) ccw
  arc A427 (29.7434, 54.4322) -> (29.7942, 54.4322) centre (29.7688, 54.4322) ccw
  line L125 (24.8158, 53.6758) -> (24.8158, 53.9355)
  line L126 (24.8158, 52.5018) -> (25.9842, 52.8913)
  arc A428 (40.0812, 9.2004) -> (40.0304, 9.2004) centre (40.0558, 9.2004) ccw
  arc A429 (25.9922, 52.8672) -> (25.9762, 52.9154) centre (25.9842, 52.8913) ccw
  line L127 (40.0558, 9.2004) -> (40.0558, 9.5899)
  arc A430 (24.8078, 52.5259) -> (24.8238, 52.4777) centre (24.8158, 52.5018) ccw
  arc A431 (24.8158, 53.8311) -> (24.8158, 53.7803) centre (24.8158, 53.8057) ccw
  arc A432 (29.8196, 28.2504) -> (29.7688, 28.2504) centre (29.7942, 28.2504) ccw
  arc A433 (30.9495, 53.8399) -> (30.9249, 53.8843) centre (30.9372, 53.8621) ccw
  line L128 (30.0934, 55.0813) -> (30.6126, 55.0813)
  line L129 (29.7688, 54.4322) -> (29.7688, 54.7567)
  arc A434 (30.0934, 55.0559) -> (30.0934, 55.1067) centre (30.0934, 55.0813) ccw
  arc A435 (41.1988, 9.2004) -> (41.2496, 9.2004) centre (41.2242, 9.2004) ccw
  arc A436 (25.9588, 53.6758) -> (26.0096, 53.6758) centre (25.9842, 53.6758) ccw
  arc A437 (40.0558, 10.8345) -> (40.0558, 10.7837) centre (40.0558, 10.8091) ccw
  arc A438 (29.7688, 54.4576) -> (29.7688, 54.4068) centre (29.7688, 54.4322) ccw
  line L130 (25.9842, 54.4336) -> (24.8158, 54.4336)
  arc A439 (29.7565, 53.2352) -> (29.7811, 53.1908) centre (29.7688, 53.213) ccw
  arc A440 (27.2622, 30.7184) -> (27.2462, 30.7666) centre (27.2542, 30.7425) ccw
  arc A441 (37.1475, 28.6724) -> (37.0967, 28.6724) centre (37.1221, 28.6724) ccw
  arc A442 (40.9646, 8.9408) -> (41.2242, 9.2004) centre (40.9646, 9.2004) ccw
  arc A443 (40.8996, 12.0029) -> (40.8996, 12.0537) centre (40.8996, 12.0283) ccw
  arc A444 (40.8996, 12.0537) -> (40.8996, 12.0029) centre (40.8996, 12.0283) ccw
  arc A445 (40.0558, 11.4046) -> (40.0558, 11.3538) centre (40.0558, 11.3792) ccw
  arc A446 (40.0304, 9.2004) -> (40.0812, 9.2004) centre (40.0558, 9.2004) ccw
  arc A447 (40.3804, 12.0283) -> (40.0558, 11.7037) centre (40.3804, 11.7037) ccw
  arc A448 (41.2365, 10.7869) -> (41.2119, 10.8313) centre (41.2242, 10.8091) ccw
  arc A449 (40.6005, 9.5899) -> (40.5497, 9.5899) centre (40.5751, 9.5899) ccw
  arc A450 (40.0435, 10.1822) -> (40.0681, 10.1378) centre (40.0558, 10.16) ccw
  arc A451 (40.0304, 11.3792) -> (40.0812, 11.3792) centre (40.0558, 11.3792) ccw
  arc A452 (41.2242, 11.7037) -> (40.8996, 12.0283) centre (40.8996, 11.7037) ccw
  arc A453 (41.2242, 11.3538) -> (41.2242, 11.4046) centre (41.2242, 11.3792) ccw
  arc A454 (40.0558, 10.1854) -> (40.0558, 10.1346) centre (40.0558, 10.16) ccw
  arc A455 (41.1988, 11.7037) -> (41.2496, 11.7037) centre (41.2242, 11.7037) ccw
  line L131 (30.2881, 52.6429) -> (30.9372, 52.6429)
  line L132 (41.2242, 11.7037) -> (41.2242, 11.3792)
  arc A456 (30.2881, 52.6683) -> (30.2881, 52.6175) centre (30.2881, 52.6429) ccw
  arc A457 (41.2242, 10.1346) -> (41.2242, 10.1854) centre (41.2242, 10.16) ccw
  arc A458 (30.9118, 52.2534) -> (30.9626, 52.2534) centre (30.9372, 52.2534) ccw
  line L133 (30.6776, 51.9938) -> (30.0284, 51.9938)
  arc A459 (41.2496, 11.7037) -> (41.1988, 11.7037) centre (41.2242, 11.7037) ccw
  arc A460 (41.2242, 9.5645) -> (41.2242, 9.6153) centre (41.2242, 9.5899) ccw
  arc A461 (40.0812, 11.7037) -> (40.0304, 11.7037) centre (40.0558, 11.7037) ccw
  arc A462 (30.9626, 52.6429) -> (30.9118, 52.6429) centre (30.9372, 52.6429) ccw
  arc A463 (41.2242, 10.7837) -> (41.2242, 10.8345) centre (41.2242, 10.8091) ccw
  line L134 (30.2881, 52.4482) -> (30.2881, 52.6429)
  arc A464 (30.6776, 51.9938) -> (30.9372, 52.2534) centre (30.6776, 52.2534) ccw
  arc A465 (30.6776, 52.0192) -> (30.6776, 51.9684) centre (30.6776, 51.9938) ccw
  arc A466 (30.0284, 52.0192) -> (30.0284, 51.9684) centre (30.0284, 51.9938) ccw
  arc A467 (30.6776, 51.9684) -> (30.6776, 52.0192) centre (30.6776, 51.9938) ccw
  line L135 (36.0299, 1.3208) -> (36.679, 1.3208)
  arc A468 (36.329, 1.3208) -> (36.3798, 1.3208) centre (36.3544, 1.3208) ccw
  line L136 (41.2242, 10.8091) -> (40.0558, 10.8091)
  arc A469 (40.3804, 12.0537) -> (40.3804, 12.0029) centre (40.3804, 12.0283) ccw
  arc A470 (40.5497, 9.3952) -> (40.6005, 9.3952) centre (40.5751, 9.3952) ccw
  arc A471 (38.7096, 11.7037) -> (38.6588, 11.7037) centre (38.6842, 11.7037) ccw
  arc A472 (30.3135, 52.6429) -> (30.2627, 52.6429) centre (30.2881, 52.6429) ccw
  arc A473 (34.2415, 29.7698) -> (34.2086, 29.7311) centre (34.2251, 29.7505) ccw
  arc A474 (30.2627, 52.4482) -> (30.3135, 52.4482) centre (30.2881, 52.4482) ccw
  arc A475 (41.2496, 9.2004) -> (41.1988, 9.2004) centre (41.2242, 9.2004) ccw
  line L137 (40.3804, 12.0283) -> (40.8996, 12.0283)
  arc A476 (30.9372, 52.6175) -> (30.9372, 52.6683) centre (30.9372, 52.6429) ccw
  line L138 (30.9372, 52.6429) -> (30.9372, 52.2534)
  arc A477 (41.2496, 9.5899) -> (41.1988, 9.5899) centre (41.2242, 9.5899) ccw
  line L139 (41.2242, 11.3792) -> (40.0558, 11.3792)
  arc A478 (30.9626, 52.2534) -> (30.9118, 52.2534) centre (30.9372, 52.2534) ccw
  arc A479 (34.8488, 29.1987) -> (34.8996, 29.1987) centre (34.8742, 29.1987) ccw
  arc A480 (34.8996, 29.8478) -> (34.8488, 29.8478) centre (34.8742, 29.8478) ccw
  line L140 (37.4142, 27.9908) -> (36.2458, 28.3803)
  line L141 (40.5751, 9.5899) -> (41.2242, 9.5899)
  arc A481 (36.2378, 28.4044) -> (36.2538, 28.3562) centre (36.2458, 28.3803) ccw
  arc A482 (41.1988, 11.3792) -> (41.2496, 11.3792) centre (41.2242, 11.3792) ccw
  line L142 (36.2458, 28.3803) -> (37.4142, 28.7697)
  line L143 (34.8742, 29.1987) -> (34.8742, 29.8478)
  line L144 (51.1246, 29.924) -> (50.9947, 29.924)
  arc A483 (37.4062, 27.9667) -> (37.4222, 28.0149) centre (37.4142, 27.9908) ccw
  arc A484 (37.4222, 28.7456) -> (37.4062, 28.7938) centre (37.4142, 28.7697) ccw
  arc A485 (40.0558, 9.2004) -> (40.3154, 8.9408) centre (40.3154, 9.2004) ccw
  arc A486 (40.3804, 12.0029) -> (40.3804, 12.0537) centre (40.3804, 12.0283) ccw
  arc A487 (36.2538, 28.4044) -> (36.2378, 28.3562) centre (36.2458, 28.3803) ccw
  arc A488 (40.0304, 11.7037) -> (40.0812, 11.7037) centre (40.0558, 11.7037) ccw
  line L145 (37.1221, 28.6724) -> (37.1221, 28.0882)
  arc A489 (37.3888, 29.1987) -> (37.4396, 29.1987) centre (37.4142, 29.1987) ccw
  arc A490 (53.9242, 30.4038) -> (53.9242, 30.4546) centre (53.9242, 30.4292) ccw
  arc A491 (53.0804, 31.0529) -> (53.0804, 31.1037) centre (53.0804, 31.0783) ccw
  arc A492 (53.3005, 28.6399) -> (53.2497, 28.6399) centre (53.2751, 28.6399) ccw
  arc A493 (52.7435, 29.2322) -> (52.7681, 29.1878) centre (52.7558, 29.21) ccw
  arc A494 (53.8988, 30.4292) -> (53.9496, 30.4292) centre (53.9242, 30.4292) ccw
  arc A495 (52.7304, 30.7537) -> (52.7812, 30.7537) centre (52.7558, 30.7537) ccw
  arc A496 (36.7397, 29.3285) -> (36.7905, 29.3285) centre (36.7651, 29.3285) ccw
  line L146 (36.2458, 29.1987) -> (36.2458, 29.5882)
  arc A497 (52.7304, 28.2504) -> (52.7812, 28.2504) centre (52.7558, 28.2504) ccw
  arc A498 (53.0154, 28.0162) -> (53.0154, 27.9654) centre (53.0154, 27.9908) ccw
  arc A499 (53.8988, 30.7537) -> (53.9496, 30.7537) centre (53.9242, 30.7537) ccw
  arc A500 (37.3888, 29.5233) -> (37.4396, 29.5233) centre (37.4142, 29.5233) ccw
  arc A501 (53.9242, 30.7537) -> (53.5996, 31.0783) centre (53.5996, 30.7537) ccw
  arc A502 (53.5996, 31.0529) -> (53.5996, 31.1037) centre (53.5996, 31.0783) ccw
  arc A503 (52.7558, 28.2504) -> (53.0154, 27.9908) centre (53.0154, 28.2504) ccw
  arc A504 (53.0154, 27.9654) -> (53.0154, 28.0162) centre (53.0154, 27.9908) ccw
  arc A505 (52.7558, 29.2354) -> (52.7558, 29.1846) centre (52.7558, 29.21) ccw
  arc A506 (37.4396, 29.5233) -> (37.3888, 29.5233) centre (37.4142, 29.5233) ccw
  arc A507 (53.0804, 31.0783) -> (52.7558, 30.7537) centre (53.0804, 30.7537) ccw
  arc A508 (53.0804, 31.1037) -> (53.0804, 31.0529) centre (53.0804, 31.0783) ccw
  line L147 (53.9242, 30.7537) -> (53.9242, 30.4292)
  arc A509 (53.9496, 30.7537) -> (53.8988, 30.7537) centre (53.9242, 30.7537) ccw
  line L148 (51.3842, 29.2749) -> (51.3842, 29.6644)
  arc A510 (53.5996, 31.1037) -> (53.5996, 31.0529) centre (53.5996, 31.0783) ccw
  line L149 (53.9242, 28.6399) -> (53.9242, 28.2504)
  arc A511 (52.7812, 28.6399) -> (52.7304, 28.6399) centre (52.7558, 28.6399) ccw
  arc A512 (53.9365, 29.8369) -> (53.9119, 29.8813) centre (53.9242, 29.8591) ccw
  arc A513 (53.9496, 28.6399) -> (53.8988, 28.6399) centre (53.9242, 28.6399) ccw
  arc A514 (52.7812, 28.2504) -> (52.7304, 28.2504) centre (52.7558, 28.2504) ccw
  arc A515 (53.9496, 28.2504) -> (53.8988, 28.2504) centre (53.9242, 28.2504) ccw
  arc A516 (37.4142, 29.5233) -> (36.7651, 29.5233) centre (37.0896, 29.5233) ccw
  arc A517 (36.2204, 29.5882) -> (36.2712, 29.5882) centre (36.2458, 29.5882) ccw